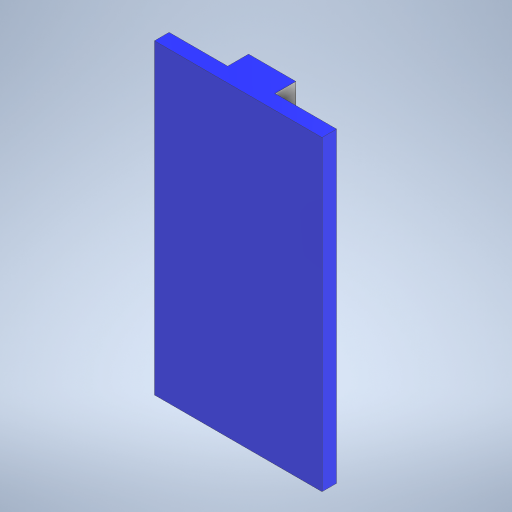
# Autodesk Inventor part: Arduino Pro Micro
Saved by Autodesk Inventor 2023.1 (Build 271208000, 208)
## iProperties
Created: 2022-10-09
Part Number: Arduino Pro Micro
Material: Generic
Document SubType Name: Modeling
Designer: Nick
Density: 1 g/cm^3
Appearance: Default
Author: Nick
Autodesk Inventor part; units mm, degrees
ref_plane "YZ Plane" through (0, 0, 0) normal (1, 0, 0) x (0, 1, 0)
ref_plane "XZ Plane" through (0, 0, 0) normal (0, 1, 0) x (-1, 0, 0)
sketch "Sketch1" plane through (0, 0, 0) normal (0, 0, 1) x (1, 0, 0)
  line L0 (0, 0) -> (18.3388, 0)
  line L1 (18.3388, 0) -> (18.3388, 33.5788)
  line L2 (18.3388, 33.5788) -> (0, 33.5788)
  line L3 (0, 33.5788) -> (0, 0)
  dimension "d0" = 18.3388
  dimension "d1" = 33.5788
  constraints: 8 end point, 2 parallel, 1 horizontal, 1 perpendicular
  measures "d0" distance of L0.start L0.end
  measures "d1" distance of L0.end L1.end
extrude "Extrusion1" add sketch "Sketch1" along normal blind 3.8862
ref_plane "Work Plane1" through (0, 0, 2.2862) normal (0, 0, 1) x (1, 0, 0)
sketch "Sketch2" plane through (0, 0, 2.2862) normal (0, 0, 1) x (1, 0, 0)
  line L0 (6.4131, 34.1392) -> (11.5922, 34.1392)
  line L1 (11.5922, 34.1392) -> (11.5922, 29.707)
  line L2 (11.5922, 29.707) -> (6.4131, 29.707)
  line L3 (6.4131, 29.707) -> (6.4131, 34.1392)
  line L4 (18.3388, 0) -> (18.3388, 33.5788) projected
  line L5 (18.3388, 33.5788) -> (0, 33.5788) projected
  line L6 (0, 33.5788) -> (0, 0) projected
  line L7 (0, 0) -> (18.3388, 0) projected
  point P0 (6.4131, 33.5788)
  point P1 (11.5922, 33.5788)
  constraints: 8 end point, 2 parallel, 1 horizontal, 1 perpendicular
extrude "Extrusion2" cut sketch "Sketch2" against normal blind 25.4 contours L3 L2 L1 L5 L4 L7 L6
body "Solid1"
